z-axis spacer_v6 (Autodesk Fusion 360 design; units mm, degrees)
Autodesk Fusion 360 part; units mm, degrees
note: some values were not read from the file. Chosen so that the rebuilt part matches the saved one: which face or edge a step refers to.
sketch "Sketch1" plane through (0, 0, 0) normal (0, 1, 0) x (1, 0, 0)
  line L0 (20, 8) -> (-20, 8)
  line L1 (-20, 8) -> (-20, -8)
  line L2 (-20, -8) -> (20, -8)
  line L3 (20, -8) -> (20, 8)
  line L4 (20, 8) -> (-20, -8) construction
  line L5 (-20, 8) -> (20, -8) construction
  line L6 (-13, 11) -> (-7, 11)
  line L7 (-7, 11) -> (-7, -8)
  line L8 (-7, -8) -> (-13, -8)
  line L9 (-13, -8) -> (-13, 11)
  line L10 (0, 0) -> (0, 17.9348) construction
  line L11 (13, 11) -> (7, 11)
  line L12 (13, -8) -> (13, 11)
  line L13 (7, 11) -> (7, -8)
  line L14 (7, -8) -> (13, -8)
  dimension "d1" = 16
  dimension "d2" = 40
  dimension "d3" = 3
  dimension "d4" = 7
  dimension "d5" = 6
  constraint horizontal L0
  constraint perpendicular L0 L1
  constraint parallel L0 L2
  constraint parallel L1 L3
  constraint coincident L4 L10.start
  constraint coincident L5 L10.start
  constraint coincident L10.start origin
  constraint horizontal L6
  constraint vertical L7
  constraint horizontal L8
  constraint vertical L9
  constraint coincident L2 L7.end
  constraint vertical L10
  constraint symmetric L6.start L10 L11.start
  constraint symmetric L6.end L10 L11.end
  constraint symmetric L7.end L10 L13.end
  constraint symmetric L8.end L10 L12.start
  measures "d1" distance of L0.start L2.end
  measures "d2" distance of L1.end L2.end
  measures "d3" distance of L0 L6
  measures "d4" distance of L7 L10
  measures "d5" distance of L6.start L6.end
extrude "Extrude1" add sketch "Sketch1" along normal blind 6 draft -1 contours L0 L2 L12 L13 L14 | L0 L11 L12 L13 | L0 L2 L7 L8 L9 | L0 L6 L7 L9 makes body 1 at (-9, 0, 1.6667) makes body 2 at (9, 0, -4.6667)
extrude "Extrude2" add sketch "Sketch1" against normal blind 16 contours L0 L2 L3 L12 | L0 L2 L12 L13 L14 | L0 L2 L7 L13 | L0 L2 L7 L8 L9 | L0 L1 L2 L9 bodies 1 2
chamfer "Chamfer1" distance 16 angle 45 1 edges at (-20, -16, 0) measured on face at (-6.6667, -16, -2.6667) on bodies 1
fillet "Fillet1" radius 1 4 edges at (-20, -0.0016, -8) (-20, -0.0032, 0) (-20, 0, 0) (-20, -0.0016, 8) on bodies 1
equation "d8 = -offset"
equation "offset = 16 mm"
equation "d11 = offset"
